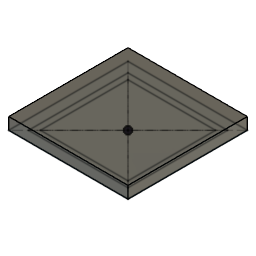
Tapa_ (Autodesk Fusion 360 design; units mm, degrees)
Autodesk Fusion 360 part; units mm, degrees
sketch "Boceto1" plane through (0, 0, 0) normal (0, 0, 1) x (1, 0, 0)
  line L0 (15, 15) -> (-15, 15)
  line L1 (-15, 15) -> (-15, -15)
  line L2 (-15, -15) -> (15, -15)
  line L3 (15, -15) -> (15, 15)
  line L4 (15, 15) -> (-15, -15) construction
  line L5 (-15, 15) -> (15, -15) construction
  line L6 (12.5, 12.5) -> (-12.5, 12.5)
  line L7 (-12.5, 12.5) -> (-12.5, -12.5)
  line L8 (-12.5, -12.5) -> (12.5, -12.5)
  line L9 (12.5, -12.5) -> (12.5, 12.5)
  line L10 (12.5, 12.5) -> (-12.5, -12.5) construction
  line L11 (-12.5, 12.5) -> (12.5, -12.5) construction
  line L12 (11, -11) -> (-11, -11)
  line L13 (-11, -11) -> (-11, 11)
  line L14 (-11, 11) -> (11, 11)
  line L15 (11, 11) -> (11, -11)
  line L16 (11, -11) -> (-11, 11) construction
  line L17 (-11, -11) -> (11, 11) construction
  dimension "d1" = 30
  dimension "d2" = 30
  dimension "d3" = 25
  dimension "d4" = 25
  dimension "d7" = 22
  dimension "d8" = 22
  constraint horizontal L0
  constraint perpendicular L0 L1
  constraint parallel L0 L2
  constraint parallel L1 L3
  constraint coincident L4 origin
  constraint coincident L5 origin
  constraint horizontal L6
  constraint perpendicular L6 L7
  constraint parallel L6 L8
  constraint parallel L7 L9
  constraint coincident L10 origin
  constraint coincident L11 origin
  constraint horizontal L12
  constraint perpendicular L12 L13
  constraint parallel L12 L14
  constraint parallel L13 L15
  constraint coincident L16 origin
  constraint coincident L17 origin
  measures "d1" distance of L0.end L1.end
  measures "d2" distance of L1.end L2.end
  measures "d3" distance of L6.end L7.end
  measures "d4" distance of L7.end L8.end
  measures "d7" distance of L12.end L13.end
  measures "d8" distance of L12.start L12.end
extrude "Extruir1" add sketch "Boceto1" along normal blind 3 contours L0 L1 L2 L3 | L6 L7 L8 L9 | L12 L13 L14 L15 makes body 1
extrude "Extruir2" add sketch "Boceto1" against normal blind 2 separate body contours L6 L7 L8 L9 makes body 2
combine "Combinar1" operation add target body 2 tool bodies 1
